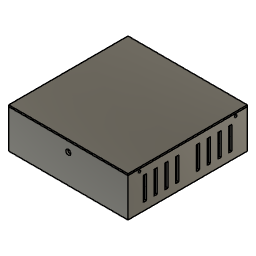
box sensors (Autodesk Fusion 360 design; units mm, degrees)
Autodesk Fusion 360 part; units mm, degrees
sketch "Boceto1" plane through (0, 0, 0) normal (0, 0, 1) x (1, 0, 0)
  line L0 (75, 75) -> (-75, 75)
  line L1 (-75, 75) -> (-75, -75)
  line L2 (-75, -75) -> (75, -75)
  line L3 (75, -75) -> (75, 75)
  line L4 (75, 75) -> (-75, -75) construction
  line L5 (-75, 75) -> (75, -75) construction
  line L6 (-77.5, -77.5) -> (77.5, -77.5)
  line L7 (77.5, -77.5) -> (77.5, 77.5)
  line L8 (77.5, 77.5) -> (-77.5, 77.5)
  line L9 (-77.5, 77.5) -> (-77.5, -77.5)
  line L10 (-75, 75) -> (-70, 75)
  line L11 (-70, 75) -> (-70, 69.5)
  line L12 (-70, 69.5) -> (-75, 69.5)
  line L13 (-75, 69.5) -> (-75, 75)
  circle A0 centre (-72.5, 72.25) radius 1.6
  line L14 (-72.5, 75) -> (-72.5, 69.5) construction
  line L15 (-75, 72.25) -> (-70, 72.25) construction
  line L16 (0, 75) -> (0, -75) construction
  line L17 (75, 0) -> (-75, 0) construction
  line L18 (70, 69.5) -> (75, 69.5)
  line L19 (70, 75) -> (70, 69.5)
  circle A1 centre (72.5, 72.25) radius 1.6
  line L20 (-70, -69.5) -> (-75, -69.5)
  line L21 (-70, -75) -> (-70, -69.5)
  circle A2 centre (-72.5, -72.25) radius 1.6
  line L22 (70, -75) -> (70, -69.5)
  line L23 (70, -69.5) -> (75, -69.5)
  circle A3 centre (72.5, -72.25) radius 1.6
  point P0 (-72.5, 72.25)
  dimension "d1" = 150
  dimension "d2" = 150
  dimension "d3" = 2.5
  dimension "d4" = 5
  dimension "d5" = 5.5
  dimension "d6" = 3.2
  constraint horizontal L0
  constraint perpendicular L0 L1
  constraint parallel L0 L2
  constraint parallel L1 L3
  constraint coincident L4 origin
  constraint coincident L5 origin
  constraint horizontal L10
  constraint vertical L11
  constraint horizontal L12
  constraint vertical L13
  constraint coincident L0.end L1.start
  constraint midpoint L10 L14.start
  constraint midpoint L12 L14.end
  constraint midpoint L13 L15.start
  constraint midpoint L11 L15.end
  constraint midpoint L14 P0
  constraint coincident P0 A0.centre
  constraint midpoint L0 L16.start
  constraint midpoint L2 L16.end
  constraint midpoint L3 L17.start
  constraint midpoint L1 L17.end
  constraint symmetric L10.end L16 L19.start
  constraint symmetric L11.end L16 L18.start
  constraint symmetric L12.end L16 L18.end
  constraint symmetric A0 L16 A1
  constraint symmetric L10.end L17 L21.start
  constraint symmetric L11.end L17 L20.start
  constraint symmetric L12.end L17 L20.end
  constraint symmetric A0 L17 A2
  constraint symmetric L17 L18.start L22.end
  constraint symmetric L17 L18.end L23.end
  constraint symmetric L17 L19.start L22.start
  constraint symmetric L17 A1 A3
  measures "d1" distance of L1 L3
  measures "d2" distance of L0 L2
  measures "d4" distance of L1 L11
  measures "d5" distance of L10 L12
  measures "d6" diameter of A0
extrude "Extruir1" add sketch "Boceto1" along normal blind 2 contours L0 L3 L18 L19 | L0 L1 L2 L3 L11 L12 L18 L19 L20 L21 L22 L23 | L0 L1 L10 L11 L12 L13 | L2 L3 L22 L23 | L1 L2 L20 L21 | L6 L7 L8 L9 | A0 | A1 | A2 | A3 makes body 1
extrude "Extruir2" add sketch "Boceto1" along normal blind 25 contours L0 L3 L18 L19 | L0 L1 L10 L11 L12 L13 | L2 L3 L22 L23 | L1 L2 L20 L21 bodies 1
extrude "Extruir3" add sketch "Boceto1" along normal blind 50 contours L6 L7 L8 L9 bodies 1
ref_plane "PlanoDeObra1" through (-77.5, 0, 25) normal (-1, 0, 0) x (0, -1, 0)
sketch "Boceto2" plane through (-77.5, 0, 0) normal (-1, 0, 0) x (0, -1, 0)
  line L0 (-77.5, 50) -> (77.5, 50) construction
  line L1 (77.5, 50) -> (77.5, 0) construction
  line L2 (77.5, 0) -> (-77.5, 0) construction
  line L3 (-77.5, 0) -> (-77.5, 50) construction
  line L4 (-67.5, 40) -> (67.5, 40)
  line L5 (67.5, 40) -> (67.5, 10)
  line L6 (67.5, 10) -> (-67.5, 10)
  line L7 (-67.5, 10) -> (-67.5, 40)
  line L8 (-57.5, 40) -> (-57.5, 10)
  line L9 (-53.5, 40) -> (-53.5, 10)
  line L10 (-43.5, 40) -> (-43.5, 10)
  line L11 (-39.5, 40) -> (-39.5, 10)
  line L12 (-29.5, 40) -> (-29.5, 10)
  line L13 (-25.5, 40) -> (-25.5, 10)
  line L14 (-15.5, 40) -> (-15.5, 10)
  line L15 (-11.5, 40) -> (-11.5, 10)
  line L16 (0, 40) -> (0, 10) construction
  line L17 (57.5, 40) -> (57.5, 10)
  line L18 (53.5, 40) -> (53.5, 10)
  line L19 (43.5, 40) -> (43.5, 10)
  line L20 (39.5, 40) -> (39.5, 10)
  line L21 (29.5, 40) -> (29.5, 10)
  line L22 (25.5, 40) -> (25.5, 10)
  line L23 (15.5, 40) -> (15.5, 10)
  line L24 (11.5, 40) -> (11.5, 10)
  point P0 (-77.5, 50)
  point P1 (77.5, 0)
  dimension "d14" = 10
  dimension "d15" = 10
  dimension "d16" = 4
  dimension "d17" = 10
  dimension "d18" = 4
  dimension "d19" = 10
  dimension "d20" = 4
  dimension "d21" = 10
  dimension "d22" = 4
  constraint horizontal L0
  constraint vertical L1
  constraint horizontal L2
  constraint vertical L3
  constraint coincident P0 L0.start
  constraint coincident P1 L1.end
  constraint coincident L4 L8.start
  constraint coincident L6 L8.end
  constraint perpendicular L6 L8
  constraint coincident L4 L9.start
  constraint coincident L6 L9.end
  constraint perpendicular L6 L9
  constraint coincident L6 L10.end
  constraint perpendicular L6 L10
  constraint coincident L4 L11.start
  constraint coincident L6 L11.end
  constraint perpendicular L6 L11
  constraint coincident L4 L12.start
  constraint coincident L6 L12.end
  constraint perpendicular L6 L12
  constraint coincident L4 L13.start
  constraint coincident L6 L13.end
  constraint perpendicular L4 L13
  constraint coincident L4 L14.start
  constraint coincident L6 L14.end
  constraint perpendicular L6 L14
  constraint coincident L4 L15.start
  constraint coincident L6 L15.end
  constraint perpendicular L6 L15
  constraint midpoint L4 L16.start
  constraint midpoint L6 L16.end
  constraint symmetric L8.start L16 L17.start
  constraint symmetric L8.end L16 L17.end
  constraint symmetric L9.start L16 L18.start
  constraint symmetric L9.end L16 L18.end
  constraint symmetric L10.start L16 L19.start
  constraint symmetric L10.end L16 L19.end
  constraint symmetric L11.start L16 L20.start
  constraint symmetric L11.end L16 L20.end
  constraint symmetric L12.start L16 L21.start
  constraint symmetric L12.end L16 L21.end
  constraint symmetric L13.start L16 L22.start
  constraint symmetric L13.end L16 L22.end
  constraint symmetric L14.start L16 L23.start
  constraint symmetric L14.end L16 L23.end
  constraint symmetric L15.start L16 L24.start
  constraint symmetric L15.end L16 L24.end
  measures "d15" distance of L7 L8
  measures "d16" distance of L8 L9
  measures "d17" distance of L9 L10
  measures "d18" distance of L10 L11
  measures "d19" distance of L11 L12
  measures "d20" distance of L12 L13
  measures "d21" distance of L13 L14
  measures "d22" distance of L14 L15
extrude "Extruir4" cut sketch "Boceto2" against normal blind 300 contours L4 L6 L8 L9 | L4 L6 L10 L11 | L4 L6 L12 L13 | L4 L6 L14 L15 | L4 L6 L23 L24 | L4 L6 L21 L22 | L4 L6 L19 L20 | L4 L6 L17 L18 bodies 1
ref_plane "PlanoDeObra2" through (0, -77.5, 25) normal (0, -1, 0) x (1, 0, 0)
sketch "Boceto3" plane through (0, -77.5, 0) normal (0, -1, 0) x (-1, 0, 0)
  line L0 (77.5, -50) -> (-77.5, -50) construction
  line L1 (-77.5, -50) -> (-77.5, 0) construction
  line L2 (-77.5, 0) -> (77.5, 0) construction
  line L3 (77.5, 0) -> (77.5, -50) construction
  line L4 (77.5, -25) -> (-77.5, -25) construction
  line L5 (0, -50) -> (0, -25) construction
  line L6 (77.5, -37.5) -> (-77.5, -37.5) construction
  circle A0 centre (0, -37.5) radius 3.25
  point P0 (77.5, -50)
  point P1 (-77.5, 0)
  point P2 (0, -37.5)
  dimension "d26" = 12.5
  dimension "d27" = 6.5
  constraint horizontal L0
  constraint vertical L1
  constraint horizontal L2
  constraint vertical L3
  constraint coincident P0 L0.start
  constraint coincident P1 L1.end
  constraint midpoint L3 L4.start
  constraint midpoint L1 L4.end
  constraint midpoint L0 L5.start
  constraint midpoint L4 L5.end
  constraint coincident L3 L6.start
  constraint coincident L1 L6.end
  constraint perpendicular L1 L6
  constraint midpoint L5 P2
  constraint coincident P2 A0.centre
  measures "d26" distance of L4 L6
  measures "d27" diameter of A0
extrude "Extruir5" cut sketch "Boceto3" against normal blind 200 bodies 1
ref_plane "PlanoDeObra3" through (72.5, 72.25, 25) normal (0, 0, 1) x (1, 0, 0)
sketch "Boceto4" plane through (0, 0, 25) normal (0, 0, 1) x (1, 0, 0)
  line L0 (-75, 75) -> (75, 75)
  line L1 (75, 75) -> (75, -75)
  line L2 (75, -75) -> (-75, -75)
  line L3 (-75, -75) -> (-75, 75)
  line L4 (0, 75) -> (0, -75) construction
  line L5 (75, 0) -> (-75, 0) construction
  line L6 (-75, 75) -> (-70, 75)
  line L7 (-70, 75) -> (-70, 69.5) construction
  line L8 (-70, 69.5) -> (-75, 69.5) construction
  line L9 (-75, 69.5) -> (-75, 75)
  line L10 (-72.5, 75) -> (-72.5, 69.5) construction
  line L11 (-70, 72.25) -> (-75, 72.25) construction
  circle A0 centre (-72.5, 72.25) radius 1.6
  circle A1 centre (72.5, 72.25) radius 1.6
  circle A2 centre (-72.5, -72.25) radius 1.6
  circle A3 centre (72.5, -72.25) radius 1.6
  line L12 (-63, 73) -> (-11, 73)
  line L13 (-11, 73) -> (-11, 33)
  line L14 (-11, 33) -> (-63, 33)
  line L15 (-63, 33) -> (-63, 73)
  line L16 (-9, 75) -> (-9, 31)
  line L17 (-9, 31) -> (-65, 31)
  line L18 (-65, 31) -> (-65, 75)
  line L19 (-65, 75) -> (-9, 75)
  line L20 (-65, 75) -> (-65, -75) construction
  point P0 (-75, 75)
  point P1 (75, -75)
  point P2 (-70, 69.5)
  point P3 (-72.5, 72.25)
  dimension "d31" = 3.2
  dimension "d32" = 52
  dimension "d33" = 40
  dimension "d34" = -2
  dimension "d35" = 10
  constraint horizontal L0
  constraint vertical L1
  constraint horizontal L2
  constraint vertical L3
  constraint coincident P0 L0.start
  constraint coincident P1 L1.end
  constraint midpoint L0 L4.start
  constraint midpoint L2 L4.end
  constraint midpoint L1 L5.start
  constraint midpoint L3 L5.end
  constraint horizontal L6
  constraint vertical L7
  constraint horizontal L8
  constraint vertical L9
  constraint coincident P2 L7.end
  constraint midpoint L6 L10.start
  constraint midpoint L8 L10.end
  constraint midpoint L7 L11.start
  constraint midpoint L9 L11.end
  constraint midpoint L10 P3
  constraint coincident P3 A0.centre
  constraint symmetric L4 A0 A1
  constraint symmetric L5 A0 A2
  constraint symmetric L5 A1 A3
  constraint horizontal L12
  constraint vertical L13
  constraint horizontal L14
  constraint vertical L15
  constraint coincident L0 L18.end
  constraint coincident L2 L20.end
  constraint perpendicular L2 L20
  constraint coincident L18.end L19.start
  measures "d31" diameter of A0
  measures "d32" distance of L12.start L12.end
  measures "d33" distance of L12.start L14.end
  measures "d35" distance of L3 L20
extrude "Extruir6" add sketch "Boceto4" along normal blind 2 separate body contours L0 L1 L2 L3 L6 L9 L16 L17 L18 | L0 L16 L17 L18 L19 | L12 L13 L14 L15 makes body 2
extrude "Extruir8" add sketch "Boceto4" along normal blind 5 contours L0 L16 L17 L18 L19 bodies 2
ref_plane "PlanoDeObra4" through (0, 77.5, 25) normal (0, 1, 0) x (-1, 0, 0)
sketch "Boceto6" plane through (0, 77.5, 0) normal (0, 1, 0) x (1, 0, 0)
  line L0 (-9, -47.861) -> (-11, -47.861) construction
  line L1 (-11, -47.861) -> (-11, -26.961) construction
  line L2 (-11, -26.961) -> (39, -26.961) construction
  line L3 (-9, -27) -> (-9, -47.861) construction
  line L4 (-11, -47.861) -> (-61, -47.861) construction
  line L5 (-61, -47.861) -> (-61, -26.961) construction
  line L6 (-61, -26.961) -> (-11, -26.961) construction
  line L7 (-11, -26.961) -> (-11, -47.861) construction
  line L8 (-61, -37.411) -> (-11, -37.411) construction
  line L9 (-46.8, -47.8805) -> (-46.8, -26.9414) construction
  line L10 (-9, -30) -> (-65, -30)
  circle A0 centre (-46.8, -37.411) radius 10.45
  circle A1 centre (-46.8, -37.411) radius 7.45
  line L11 (-44.502, -44.4977) -> (-43.9775, -47.4726)
  line L12 (-49.098, -44.4977) -> (-49.6225, -47.4726)
  line L13 (-44.502, -30.3242) -> (-43.9775, -27.3494)
  line L14 (-49.098, -30.3242) -> (-49.6225, -27.3494)
  line L15 (-39.5704, -39.2096) -> (-36.6109, -39.7315)
  line L16 (-39.5704, -35.6123) -> (-36.6109, -35.0905)
  line L17 (-54.0296, -39.2096) -> (-56.9891, -39.7315)
  line L18 (-54.0296, -35.6123) -> (-56.9891, -35.0905)
  point P0 (-9, -27)
  point P1 (-46.8, -37.411)
  dimension "d43" = 20.9
  dimension "d44" = 2
  dimension "d45" = 50
  dimension "d54" = 3.039
  dimension "d66" = 35.8
  dimension "d67" = -3
  dimension "d68" = 10
  dimension "d69" = 7.0867
  dimension "d70" = 10
  dimension "d71" = 7.2296
  constraint horizontal L0
  constraint vertical L1
  constraint horizontal L2
  constraint vertical L3
  constraint coincident P0 L3.start
  constraint horizontal L4
  constraint vertical L5
  constraint horizontal L6
  constraint vertical L7
  constraint coincident L1.end L2.start
  constraint coincident L0.end L1.start
  constraint midpoint L5 L8.start
  constraint midpoint L7 L8.end
  constraint perpendicular L6 L9
  constraint midpoint L9 P1
  constraint coincident P1 A0.centre
  constraint tangent L4 A0
  constraint tangent L6 A0
  constraint coincident A1 L11.start
  constraint coincident A0 L11.end
  constraint symmetric L9 L11.start L12.start
  constraint symmetric L9 L11.end L12.end
  constraint symmetric L8 L11.start L13.start
  constraint symmetric L8 L11.end L13.end
  constraint symmetric L8 L12.start L14.start
  constraint symmetric L8 L12.end L14.end
  constraint coincident A1 L15.start
  constraint coincident A0 L15.end
  constraint symmetric L8 L15.start L16.start
  constraint symmetric L8 L15.end L16.end
  constraint symmetric L9 L15.start L17.start
  constraint symmetric L9 L15.end L17.end
  constraint symmetric L9 L16.start L18.start
  constraint symmetric L9 L16.end L18.end
  measures "d43" distance of L0 L2
  measures "d44" distance of L1 L3
  measures "d45" distance of L5 L7
  measures "d54" distance of L6 L10
  measures "d66" distance of L1 L9
  measures "d68" angle of L9 L11
  measures "d69" distance of L8 L11.start
  measures "d70" angle of L8 L15
  measures "d71" distance of L9 L15.start
extrude "Extruir9" cut sketch "Boceto6" against normal blind 9 contours L10 A0 A1 L13 L16 | L10 A0 L13 | L10 A0 L14 | A0 A1 L11 L15 | L10 A0 A1 L14 L18 | A0 A1 L12 L17 bodies 1 2
fillet "Empalme1" radius 1 17 edges at (-56.9891, 76.25, 39.7315) (-43.9775, 76.25, 27.3494) (-39.5704, 76.25, 39.2096) (-44.502, 76.25, 44.4977) (-49.6225, 76.25, 27.3494) (-54.0296, 76.25, 39.2096) (-49.098, 76.25, 44.4977) (-36.6109, 76.25, 39.7315) (-39.5704, 76.25, 35.6123) (-43.9775, 76.25, 47.4726) (-56.9891, 76.25, 35.0905) (-36.6109, 76.25, 35.0905) (-49.098, 76.25, 30.3242) (-54.0296, 76.25, 35.6123) (-49.6225, 76.25, 47.4726) (-43.9775, 74, 27.3494) (-49.6225, 74, 27.3494) on bodies 1 2
ref_plane "PlanoDeObra5" through (0, 0, 50) normal (0, 0, 1) x (1, 0, 0)
sketch "Boceto7" plane through (0, 0, 50) normal (0, 0, 1) x (1, 0, 0)
  line L0 (-77.5, 77.5) -> (77.5, 77.5)
  line L1 (77.5, 77.5) -> (77.5, -77.5)
  line L2 (77.5, -77.5) -> (-77.5, -77.5)
  line L3 (-77.5, -77.5) -> (-77.5, 77.5)
  line L4 (-75, 75) -> (75, 75)
  line L5 (75, 75) -> (75, -75)
  line L6 (75, -75) -> (-75, -75)
  line L7 (-75, -75) -> (-75, 75)
  line L8 (72.5, -72.5) -> (-72.5, -72.5)
  line L9 (-72.5, -72.5) -> (-72.5, 72.5)
  line L10 (-72.5, 72.5) -> (72.5, 72.5)
  line L11 (72.5, 72.5) -> (72.5, -72.5)
  point P0 (-77.5, 77.5)
  point P1 (77.5, -77.5)
  point P2 (75, -75)
  point P3 (-75, 75)
  dimension "d77" = 2.5
  constraint horizontal L0
  constraint vertical L1
  constraint horizontal L2
  constraint vertical L3
  constraint coincident P0 L0.start
  constraint coincident P1 L1.end
  constraint horizontal L4
  constraint vertical L5
  constraint horizontal L6
  constraint vertical L7
  constraint coincident P2 L5.end
  constraint coincident P3 L4.start
extrude "Extruir10" add sketch "Boceto7" against normal blind 10 separate body contours L4 L5 L6 L7 makes body 3
extrude "Extruir11" add sketch "Boceto7" along normal blind 2 contours L0 L1 L2 L3 | L4 L5 L6 L7 | L8 L9 L10 L11 bodies 3
sketch "Boceto8" plane through (-77.5, 0, 0) normal (-1, 0, 0) x (0, -1, 0)
  line L0 (77.5, 50) -> (-77.5, 50) construction
  line L1 (-77.5, 50) -> (-77.5, 44) construction
  line L2 (-77.5, 44) -> (77.5, 44) construction
  line L3 (77.5, 44) -> (77.5, 50) construction
  line L4 (-77.5, 47) -> (77.5, 47) construction
  circle A0 centre (-62.5, 47) radius 1.6
  line L5 (0, 50) -> (0, 44) construction
  circle A1 centre (62.5, 47) radius 1.6
  point P0 (77.5, 50)
  point P1 (-77.5, 50)
  dimension "d82" = 6
  dimension "d83" = 3.2
  dimension "d84" = 15
  constraint horizontal L0
  constraint vertical L1
  constraint horizontal L2
  constraint vertical L3
  constraint coincident P0 L0.start
  constraint coincident P1 L0.end
  constraint midpoint L1 L4.start
  constraint midpoint L3 L4.end
  constraint coincident L4 A0.centre
  constraint midpoint L0 L5.start
  constraint midpoint L2 L5.end
  constraint symmetric A0 L5 A1
  measures "d82" distance of L0 L2
  measures "d83" diameter of A0
  measures "d84" distance of L4.start A0.centre
extrude "Extruir12" cut sketch "Boceto8" against normal blind 200 bodies 1 3
